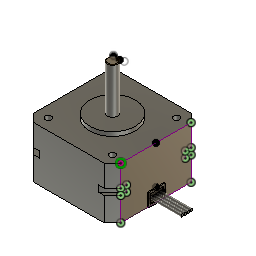
Dual Bondtech extruder with mosquito v2 (Autodesk Fusion 360 archive; units mm, degrees)
design "motor, stepper, NEMA 17, 25mm pancake"
Autodesk Fusion 360 part; units mm, degrees
sketch "Sketch1" plane through (0, 0, 0) normal (0, 0, 1) x (1, 0, 0) in component "NEMA 17 Stepper (Steppermotor 17HM19-2004S)"
  line L0 (36.7456, 89.6744) -> (102.2059, 89.6744) construction
  line L1 (102.2059, 89.6744) -> (102.2059, 33.5078) construction
  circle A0 centre (102.2059, 89.6744) radius 11
  circle A1 centre (86.7059, 74.1744) radius 1.5
  circle A2 centre (86.7059, 105.1744) radius 1.5
  circle A3 centre (117.7059, 74.1744) radius 1.5
  circle A4 centre (117.7059, 105.1744) radius 1.5
  line L2 (81.2059, 110.6744) -> (123.2059, 110.6744)
  line L3 (123.2059, 110.6744) -> (123.2059, 68.6744)
  line L4 (123.2059, 68.6744) -> (81.2059, 68.6744)
  line L5 (81.2059, 68.6744) -> (81.2059, 110.6744)
  circle A5 centre (102.2059, 89.6744) radius 2.5
  dimension "d18" = 22
  dimension "d19" = 3
  dimension "d20" = 15.5
  dimension "d21" = 15.5
  dimension "d22" = 42
  dimension "d23" = 21
  dimension "d24" = 42
  dimension "d25" = 21
  dimension "d26" = 5
  constraint horizontal L0
  constraint vertical L1
  constraint coincident L0.end L1.start
  constraint symmetric L0 A1 A2
  constraint symmetric L1 A1 A3
  constraint symmetric L1 A2 A4
  constraint horizontal L2
  constraint vertical L3
  constraint horizontal L4
  constraint vertical L5
  constraint concentric A0 A5
  measures "d18" diameter of A0
  measures "d19" diameter of A1
  measures "d20" distance of L0 A1.centre
  measures "d21" distance of L1 A1.centre
  measures "d22" distance of L3 L5
  measures "d23" distance of L1 L3
  measures "d24" distance of L2 L4
  measures "d25" distance of L0 L4
  measures "d26" diameter of A5
extrude "Extrude4" add sketch "Sketch1" along normal blind -25 and the other way blind 13.5 contours A0 | L2 L3 L4 L5 makes body 1 in component "NEMA 17 Stepper (Steppermotor 17HM19-2004S)"
extrude "Extrude1" add sketch "Sketch1" against normal blind 10.5 separate body contours A0 | L2 L3 L4 L5 | A5 makes body 2 in component "NEMA 17 Stepper (Steppermotor 17HM19-2004S)"
extrude "Extrude2" add sketch "Sketch1" along normal blind 24 contours A5 bodies 2 in component "NEMA 17 Stepper (Steppermotor 17HM19-2004S)"
extrude "Extrude3" add sketch "Sketch1" along normal blind 2 contours A0 bodies 2 in component "NEMA 17 Stepper (Steppermotor 17HM19-2004S)"
chamfer "Chamfer1" distance 4 angle 45 8 edges at (123.2059, 110.6744, -5.25) (81.2059, 110.6744, -5.25) (123.2059, 68.6744, -5.25) (81.2059, 68.6744, -5.25) (123.2059, 110.6744, -19.25) (81.2059, 110.6744, -19.25) (123.2059, 68.6744, -19.25) (81.2059, 68.6744, -19.25) on bodies 1 2 in component "NEMA 17 Stepper (Steppermotor 17HM19-2004S)"
sketch "Sketch3" plane through (0, 0, -13.5) normal (0, 0, 1) x (-1, 0, 0) in component "NEMA 17 Stepper (Steppermotor 17HM19-2004S)"
  circle A0 centre (-102.2059, -89.6744) radius 2.5
  circle A1 centre (-117.7059, -105.1744) radius 1.5
  circle A2 centre (-86.7059, -105.1744) radius 1.5
  circle A3 centre (-86.7059, -74.1744) radius 1.5
  circle A4 centre (-117.7059, -74.1744) radius 1.5
  line L0 (-81.2059, -72.6744) -> (-85.2059, -68.6744)
  line L1 (-85.2059, -68.6744) -> (-119.2059, -68.6744)
  line L2 (-119.2059, -68.6744) -> (-123.2059, -72.6744)
  line L3 (-123.2059, -72.6744) -> (-123.2059, -106.6744)
  line L4 (-123.2059, -106.6744) -> (-119.2059, -110.6744)
  line L5 (-119.2059, -110.6744) -> (-85.2059, -110.6744)
  line L6 (-85.2059, -110.6744) -> (-81.2059, -106.6744)
  line L7 (-81.2059, -106.6744) -> (-81.2059, -72.6744)
  arc A5 (-116.4185, -68.6744) -> (-123.2059, -75.4618) centre (-84.6201, -107.2602) ccw
  line L8 (-81.2059, -103.846) -> (-88.0344, -110.6744) construction
  line L9 (-36.7456, -89.6744) -> (-102.2059, -89.6744) construction
  line L10 (-102.2059, -89.6744) -> (-102.2059, -33.5078) construction
  arc A6 (-81.2059, -75.4618) -> (-87.9933, -68.6744) centre (-119.7917, -107.2602) ccw
  arc A7 (-123.2059, -103.887) -> (-116.4185, -110.6744) centre (-84.6201, -72.0886) ccw
  arc A8 (-87.9933, -110.6744) -> (-81.2059, -103.887) centre (-119.7917, -72.0886) ccw
  dimension "d39" = 50
  dimension "d40" = 2
  constraint parallel L6 L8
  constraint coincident L5 L8.end
  constraint coincident L7 L8.start
  constraint midpoint A5.centre L8
  constraint coincident L3 A5.end
  constraint coincident L1 A5.start
  constraint symmetric A5 L10 A6
  constraint symmetric A5.end L10 A6.start
  constraint symmetric A5.start L10 A6.end
  constraint symmetric A5 L9 A7
  constraint symmetric A5.end L9 A7.start
  constraint symmetric A5.start L9 A7.end
  constraint symmetric L9 A6.end A8.start
  constraint symmetric L9 A6.start A8.end
  constraint symmetric L9 A6 A8
  measures "d39" radius of A5
  measures "d40" distance of L6 L8
extrude "Extrude5" add sketch "Sketch3" along normal blind 3.5 contours A0 | L1 L3 L5 L7 A5 A6 A7 A8 bodies 2 1 in component "NEMA 17 Stepper (Steppermotor 17HM19-2004S)"
sketch "Sketch4" plane through (0, 0, 24) normal (0, 0, 1) x (-1, 0, 0) in component "NEMA 17 Stepper (Steppermotor 17HM19-2004S)"
  circle A0 centre (-102.2059, -89.6744) radius 2.5
  line L0 (-100.7059, -91.6744) -> (-103.7059, -91.6744)
  line L1 (-100.1798, -92.1744) -> (-105.3666, -92.1744) construction
  dimension "d43" = 0.5
  constraint horizontal L0
  constraint coincident A0 L0.start
  constraint coincident A0 L0.end
  constraint horizontal L1
  constraint tangent A0 L1
  measures "d43" distance of L0 L1
extrude "Extrude6" cut sketch "Sketch4" against normal blind 15 contours A0 L0 picked at (-102.6058, -91.7388) bodies 2 in component "NEMA 17 Stepper (Steppermotor 17HM19-2004S)"
chamfer "Chamfer2" distance 0.25 angle 45 1 edges at (102.2059, 87.1744, 24) on bodies 2 in component "NEMA 17 Stepper (Steppermotor 17HM19-2004S)"
sketch "Sketch5" plane through (123.2059, 0, 0) normal (1, 0, 0) x (0, 1, 0) in component "NEMA 17 Stepper (Steppermotor 17HM19-2004S)"
  line L0 (72.6744, -13.5) -> (72.6744, -25)
  line L1 (72.6744, -25) -> (106.6744, -25)
  line L2 (106.6744, -25) -> (106.6744, -13.5)
  line L3 (106.6744, -13.5) -> (103.887, -13.5)
  line L4 (103.887, -13.5) -> (103.887, -10.5)
  line L5 (103.887, -10.5) -> (106.6744, -10.5)
  line L6 (106.6744, -10.5) -> (106.6744, 0)
  line L7 (106.6744, 0) -> (72.6744, 0)
  line L8 (72.6744, 0) -> (72.6744, -10.5)
  line L9 (72.6744, -10.5) -> (75.4618, -10.5)
  line L10 (75.4618, -10.5) -> (75.4618, -13.5)
  line L11 (75.4618, -13.5) -> (72.6744, -13.5)
  line L12 (85.6744, -18.5) -> (93.6744, -18.5)
  line L13 (93.6744, -18.5) -> (93.6744, -25)
  line L14 (93.6744, -25) -> (85.6744, -25)
  line L15 (85.6744, -25) -> (85.6744, -18.5)
  line L16 (92.6744, -24) -> (86.6744, -24)
  line L17 (86.6744, -24) -> (86.6744, -19.5)
  line L18 (86.6744, -19.5) -> (92.6744, -19.5)
  line L19 (92.6744, -19.5) -> (92.6744, -24)
  circle A0 centre (87.4244, -21.75) radius 0.625
  circle A1 centre (88.9244, -21.75) radius 0.625
  circle A2 centre (90.4244, -21.75) radius 0.625
  circle A3 centre (91.9244, -21.75) radius 0.625
  line L20 (103.887, -10.5) -> (106.6744, -10.5)
  line L21 (106.6744, -10.5) -> (106.6744, 0)
  line L22 (106.6744, 0) -> (72.6744, 0)
  line L23 (72.6744, 0) -> (72.6744, -10.5)
  line L24 (72.6744, -10.5) -> (75.4618, -10.5)
  line L25 (75.4618, -10.5) -> (75.4618, -13.5)
  line L26 (75.4618, -13.5) -> (72.6744, -13.5)
  line L27 (72.6744, -13.5) -> (72.6744, -25)
  line L28 (72.6744, -25) -> (106.6744, -25)
  line L29 (106.6744, -25) -> (106.6744, -13.5)
  line L30 (106.6744, -13.5) -> (103.887, -13.5)
  line L31 (103.887, -13.5) -> (103.887, -10.5)
  point P0 (89.6744, 0)
  point P1 (89.6744, -18.5)
  point P2 (92.6744, -21.75)
  dimension "d47" = 8
  dimension "d48" = 6.5
  dimension "d49" = 1
  dimension "d50" = 1.25
  dimension "d53" = 1.5
  dimension "d54" = 0
  dimension "d60" = 0.75
  constraint horizontal L12
  constraint vertical L13
  constraint horizontal L14
  constraint vertical L15
  constraint collinear L1 L14
  constraint midpoint L22 P0
  constraint midpoint L12 P1
  constraint vertical P0 P1
  constraint midpoint L19 P2
  constraint horizontal A0.centre P2
  measures "d47" distance of L12.start L12.end
  measures "d48" distance of L12.start L14.end
  measures "d50" diameter of A0
  measures "d60" horizontal distance of A1.centre P1
extrude "Extrude7" add sketch "Sketch5" along normal blind 0.5 contours L1 L12 L13 L14 L15 L28 bodies 2 in component "NEMA 17 Stepper (Steppermotor 17HM19-2004S)"
extrude "Extrude8" add sketch "Sketch5" along normal blind 15 contours A0 | A1 | A2 | A3 bodies 2 in component "NEMA 17 Stepper (Steppermotor 17HM19-2004S)"
component "NEMA 17 Stepper (Steppermotor 17HM19-2004S)" placed x (1, 0, 0) y (0, 1, 0) z (0, 0, 1) at (0, 0, 0)
equation "d20 = ( 31 / 2 ) * 1 mm"
equation "d21 = d20"
equation "d23 = d22 / 2"
equation "d24 = d22"
equation "d25 = d23"
equation "d33 = -body_length"
equation "d35 = body_length - 11.5 mm"
equation "d41 = body_length - 21.5 mm"
equation "body_length = 25 mm"
